Autodesk Fusion 360 part; units mm, degrees
(part 3 of 3)
  point P284 (15.4508, 47.5528)
  point P285 (-0.5155, 69.5286)
  point P286 (-5, 67.1945)
  point P287 (10.0646, 54.9663)
  point P288 (50, 67.9421)
  point P289 (39.8583, 55.4833)
  point P290 (50, 69.4421)
  point P291 (55, 67.1945)
  point P292 (43.541, 51.4226)
  point P293 (98.1857, -14.3619)
  point P294 (105.9017, -18.1636)
  point P295 (99.4427, -25.5195)
  point P296 (99.4698, -11.8417)
  point P297 (97.1866, -20.9953)
  point P298 (89.9352, -18.0941)
  point P299 (91.7173, -33.287)
  point P300 (55.3862, 7.4135)
  point P301 (56.2679, 8.627)
  point P302 (50.9017, 9.7476)
  point P303 (80.0676, 26.5576)
  point P304 (80.9017, 31.5439)
  point P305 (66.4847, 14.1828)
  point P306 (80.9017, 0)
  point P307 (52.5861, 20.5725)
  point P308 (62.958, 9.3287)
  point P309 (65.9663, 21.9758)
  point P310 (62.3607, 25.5195)
  point P311 (65.0847, 20.7623)
  point P312 (81.4942, 26.094)
  point P313 (99.9017, 12)
  point P314 (97.9017, 14)
  point P315 (89.9352, 18.0941)
  point P316 (80.9017, 0)
  point P317 (115.9017, 0)
  point P318 (75.3603, 21.7783)
  point P319 (58.477, 1.4597)
  point P320 (84.2289, 19.9482)
  point P321 (71.3525, 29.3893)
  point P322 (50, 0)
  point P323 (72.8402, 20.4942)
  point P324 (95.76, 21.4588)
  point P325 (105.9017, 7.5)
  point P326 (55.3862, -7.4135)
  point P327 (58.9194, -1.3339)
  point P328 (72.5838, -20.8761)
  point P329 (71.3525, -29.3893)
  point P330 (75.3774, -21.3186)
  point P331 (62.958, -9.3287)
  point P332 (52.5861, -20.5725)
  point P333 (105.9017, -7.5)
  point P334 (84.2289, -19.9482)
  point P335 (66.4847, -14.1828)
  point P336 (50.9017, -9.7476)
  point P337 (65.0847, -20.7623)
  point P338 (65.9663, -21.9758)
  point P339 (80.9017, -31.5439)
  point P340 (110.9017, -9.7476)
  point P341 (91.7173, 33.287)
  point P342 (100.9017, -3)
  point P343 (80.0676, -26.5576)
  point P344 (105.9017, -9)
  point P345 (95.76, -21.4588)
  point P346 (81.4942, -26.094)
  point P347 (105.9017, 9)
  point P348 (62.3607, -25.5195)
  point P349 (97.1866, 20.9953)
  point P350 (99.4427, 25.5195)
  point P351 (56.2679, -8.627)
  dimension "d15" = -5
  dimension "d17" = 360
  dimension "d19" = 360
  dimension "d22" = 360
  constraint coincident L11.start origin
  constraint coincident S5 L10.start
  constraint horizontal L11
  constraint midpoint S10.start L13
  constraint coincident S10 L15.start
  constraint midpoint S12.start L19
  constraint midpoint S6.start L21
  constraint midpoint S2.start L23
  constraint midpoint S7.start L25
  constraint midpoint S13.start L27
  constraint midpoint S18.start L33
  constraint midpoint S8.start L38
  constraint midpoint S3.start L42
  constraint midpoint S5.start L44
  constraint midpoint S4.start L46
  constraint midpoint S14.start L49
  constraint midpoint S0.start L51
  constraint midpoint S15.start L56
  constraint midpoint S1.start L58
  constraint midpoint S17.start L60
  constraint midpoint S9.start L62
  constraint midpoint S19.start L65
  constraint midpoint S16.start L68
  constraint symmetric L11.start L1 P92
  constraint symmetric L0.start L1 L29.start
  constraint symmetric L0.end L1 L29.end
  constraint symmetric L2.start L1 L54.start
  constraint symmetric L2.end L1 L41.start
  constraint symmetric L3.end L1 L40.start
  constraint symmetric L1 L5.start L30.end
  constraint symmetric L1 L5.end L53.start
  constraint symmetric L1 L6.end L32.start
  constraint symmetric L1 L7.end L31.start
  constraint symmetric L1 L8.end L30.start
  constraint symmetric L1 S0.start S32.start
  constraint symmetric L1 L12.end L36.end
  constraint symmetric L1 P0 P82
  constraint symmetric L1 P1 P76
  constraint symmetric L1 S1.start S34.start
  constraint symmetric L1 P2 P93
  constraint symmetric L1 P3 P97
  constraint symmetric L1 P4 P91
  constraint symmetric L1 S2.start S22.start
  constraint symmetric L1 P5 P72
  constraint symmetric L1 P6 P114
  constraint symmetric L1 P7 P59
  constraint symmetric L1 S3.start S27.start
  constraint symmetric L1 P8 P69
  constraint symmetric L1 P9 P78
  constraint symmetric L1 P10 P77
  constraint symmetric L1 S4.start S29.start
  constraint symmetric L1 P11 P110
  constraint symmetric L1 P12 P83
  constraint symmetric L1 P13 P89
  constraint symmetric L1 S5.start S28.start
  constraint symmetric L1 L10.end L64.end
  constraint symmetric L1 P14 P99
  constraint symmetric L1 P15 P88
  constraint symmetric L1 L10.start L64.start
  constraint symmetric L1 S6.start S21.start
  constraint symmetric L1 P16 P98
  constraint symmetric L1 P17 P70
  constraint symmetric L1 P18 P95
  constraint symmetric L1 S7.start S23.start
  constraint symmetric L1 P19 P64
  constraint symmetric L1 P20 P63
  constraint symmetric L1 P21 P67
  constraint symmetric L1 S8.start S26.start
  constraint symmetric L1 P22 P100
  constraint symmetric L1 P23 P79
  constraint symmetric L1 P24 P68
  constraint symmetric L1 S9.start S36.start
  constraint symmetric L1 P25 P75
  constraint symmetric L1 P26 P71
  constraint symmetric L1 P27 P81
  constraint symmetric L1 L11.start P92
  constraint symmetric L1 L16.end L35.end
  constraint symmetric L1 L11.end L37.end
  constraint symmetric L1 L15.end L17.end
  constraint symmetric L1 L12.start L36.start
  constraint symmetric L1 S10.start S38.start
  constraint symmetric L1 P28 P108
  constraint symmetric L1 P29 P106
  constraint symmetric L1 P30 P73
  constraint symmetric L1 S11.start S30.start
  constraint symmetric L1 P31 P112
  constraint symmetric L1 P32 P105
  constraint symmetric L1 L13.start L18.start
  constraint symmetric L1 L13.end L18.end
  constraint symmetric L1 L14.start L48.start
  constraint symmetric L1 L14.end L48.end
  constraint symmetric L1 L15.start L17.start
  constraint symmetric L1 S12.start S20.start
  constraint symmetric L1 P33 P103
  constraint symmetric L1 P34 P113
  constraint symmetric L1 P35 P102
  constraint symmetric L1 S13.start S24.start
  constraint symmetric L1 P36 P107
  constraint symmetric L1 P37 P104
  constraint symmetric L1 P38 P109
  constraint symmetric L1 S14.start S31.start
  constraint symmetric L1 P39 P65
  constraint symmetric L1 P40 P115
  constraint symmetric L1 P41 P84
  constraint symmetric L1 S15.start S33.start
  constraint symmetric L1 P42 P96
  constraint symmetric L1 P43 P111
  constraint symmetric L1 P44 P101
  constraint symmetric L1 S16.start S39.start
  constraint symmetric L1 P45 P62
  constraint symmetric L1 P46 P58
  constraint symmetric L1 P47 P74
  constraint symmetric L1 S17.start S35.start
  constraint symmetric L1 P48 P60
  constraint symmetric L1 P49 P87
  constraint symmetric L1 P50 P57
  constraint symmetric L1 S18.start S25.start
  constraint symmetric L1 P51 P86
  constraint symmetric L1 P52 P80
  constraint symmetric L1 P53 P94
  constraint symmetric L1 S19.start S37.start
  constraint symmetric L1 P54 P85
  constraint symmetric L1 P55 P66
  constraint symmetric L1 P56 P61
  constraint symmetric L1 L19.start L20.start
  constraint symmetric L1 L19.end L20.end
  constraint symmetric L1 L21.start L22.start
  constraint symmetric L1 L21.end L22.end
  constraint symmetric L1 L23.start L24.start
  constraint symmetric L1 L23.end L24.end
  constraint symmetric L1 L25.start L26.start
  constraint symmetric L1 L25.end L26.end
  constraint symmetric L1 L27.start L28.start
  constraint symmetric L1 L27.end L28.end
  constraint symmetric L1 L33.start L34.start
  constraint symmetric L1 L33.end L34.end
  constraint symmetric L1 L38.start L39.start
  constraint symmetric L1 L38.end L39.end
  constraint symmetric L1 L42.start L43.start
  constraint symmetric L1 L42.end L43.end
  constraint symmetric L1 L44.start L45.start
  constraint symmetric L1 L44.end L45.end
  constraint symmetric L1 L46.start L47.start
  constraint symmetric L1 L46.end L47.end
  constraint symmetric L1 L49.start L50.start
  constraint symmetric L1 L49.end L50.end
  constraint symmetric L1 L51.start L52.start
  constraint symmetric L1 L51.end L52.end
  constraint symmetric L1 L56.start L57.start
  constraint symmetric L1 L56.end L57.end
  constraint symmetric L1 L58.start L59.start
  constraint symmetric L1 L58.end L59.end
  constraint symmetric L1 L60.start L61.start
  constraint symmetric L1 L60.end L61.end
  constraint symmetric L1 L62.start L63.start
  constraint symmetric L1 L62.end L63.end
  constraint symmetric L1 L65.start L66.start
  constraint symmetric L1 L65.end L66.end
  constraint symmetric L1 L68.start L69.start
  constraint symmetric L1 L68.end L69.end
  constraint symmetric L11.start L0 P147
  constraint symmetric L4.end L0 L116.end
  constraint symmetric L1.start L0 L29.end
  constraint symmetric L1.end L0 L121.start
  constraint symmetric L2.end L0 L119.start
  constraint symmetric L3.end L0 L116.start
  constraint symmetric L0 L5.start L122.start
  constraint symmetric L0 L5.end L120.start
  constraint symmetric L0 L6.end L118.start
  constraint symmetric L0 L7.end L117.start
  constraint symmetric L0 L8.end L117.end
  constraint symmetric L0 S0.start S50.start
  constraint symmetric L0 L12.end L98.end
  constraint symmetric L0 P0 P149
  constraint symmetric L0 P1 P166
  constraint symmetric L0 S1.start S56.start
  constraint symmetric L0 P2 P158
  constraint symmetric L0 P3 P160
  constraint symmetric L0 P4 P171
  constraint symmetric L0 S2.start S59.start
  constraint symmetric L0 P5 P174
  constraint symmetric L0 P6 P172
  constraint symmetric L0 P7 P173
  constraint symmetric L0 S3.start S54.start
  constraint symmetric L0 P8 P145
  constraint symmetric L0 P9 P146
  constraint symmetric L0 P10 P128
  constraint symmetric L0 S4.start S52.start
  constraint symmetric L0 P11 P155
  constraint symmetric L0 P12 P162
  constraint symmetric L0 P13 P144
  constraint symmetric L0 S5.start S47.start
  constraint symmetric L0 L10.end L96.end
  constraint symmetric L0 P14 P130
  constraint symmetric L0 P15 P134
  constraint symmetric L0 L10.start L96.start
  constraint symmetric L0 S6.start S57.start
  constraint symmetric L0 P16 P132
  constraint symmetric L0 P17 P131
  constraint symmetric L0 P18 P135
  constraint symmetric L0 S7.start S58.start
  constraint symmetric L0 P19 P170
  constraint symmetric L0 P20 P123
  constraint symmetric L0 P21 P119
  constraint symmetric L0 S8.start S45.start
  constraint symmetric L0 P22 P148
  constraint symmetric L0 P23 P150
  constraint symmetric L0 P24 P151
  constraint symmetric L0 S9.start S46.start
  constraint symmetric L0 P25 P157
  constraint symmetric L0 P26 P154
  constraint symmetric L0 P27 P152
  constraint symmetric L0 L11.start P147
  constraint symmetric L0 L16.end L104.end
  constraint symmetric L0 L11.end L99.end
  constraint symmetric L0 L15.end L104.start
  constraint symmetric L0 L12.start L98.start
  constraint symmetric L0 S10.start S44.start
  constraint symmetric L0 P28 P138
  constraint symmetric L0 P29 P142
  constraint symmetric L0 P30 P136
  constraint symmetric L0 S11.start S53.start
  constraint symmetric L0 P31 P139
  constraint symmetric L0 P32 P133
  constraint symmetric L0 L13.start L83.start
  constraint symmetric L0 L13.end L83.end
  constraint symmetric L0 L14.start L106.start
  constraint symmetric L0 L14.end L106.end
  constraint symmetric L0 L15.start L105.start
  constraint symmetric L0 S12.start S41.start
  constraint symmetric L0 P33 P141
  constraint symmetric L0 P34 P164
  constraint symmetric L0 P35 P159
  constraint symmetric L0 S13.start S42.start
  constraint symmetric L0 P36 P169
  constraint symmetric L0 P37 P156
  constraint symmetric L0 P38 P165
  constraint symmetric L0 S14.start S55.start
  constraint symmetric L0 P39 P120
  constraint symmetric L0 P40 P121
  constraint symmetric L0 P41 P122
  constraint symmetric L0 S15.start S43.start
  constraint symmetric L0 P42 P126
  constraint symmetric L0 P43 P127
  constraint symmetric L0 P44 P125
  constraint symmetric L0 S16.start S48.start
  constraint symmetric L0 P45 P167
  constraint symmetric L0 P46 P168
  constraint symmetric L0 P47 P153
  constraint symmetric L0 S17.start S40.start
  constraint symmetric L0 P48 P124
  constraint symmetric L0 P49 P117
  constraint symmetric L0 P50 P116
  constraint symmetric L0 S18.start S51.start
  constraint symmetric L0 P51 P163
  constraint symmetric L0 P52 P129
  constraint symmetric L0 P53 P140
  constraint symmetric L0 S19.start S49.start
  constraint symmetric L0 P54 P143
  constraint symmetric L0 P55 P137
  constraint symmetric L0 P56 P161
  constraint symmetric L0 L19.start L77.start
  constraint symmetric L0 L19.end L77.end
  constraint symmetric L0 L21.start L80.start
  constraint symmetric L0 L21.end L80.end
  constraint symmetric L0 L23.start L103.start
  constraint symmetric L0 L23.end L103.end
  constraint symmetric L0 L25.start L74.start
  constraint symmetric L0 L25.end L74.end
  constraint symmetric L0 L27.start L78.start
  constraint symmetric L0 L27.end L78.end
  constraint symmetric L0 L33.start L82.start
  constraint symmetric L0 L33.end L82.end
  constraint symmetric L0 L38.start L84.start
  constraint symmetric L0 L38.end L84.end
  constraint symmetric L0 L42.start L88.start
  constraint symmetric L0 L42.end L88.end
  constraint symmetric L0 L44.start L85.start
  constraint symmetric L0 L44.end L85.end
  constraint symmetric L0 L46.start L100.start
  constraint symmetric L0 L46.end L100.end
  constraint symmetric L0 L49.start L75.start
  constraint symmetric L0 L49.end L75.end
  constraint symmetric L0 L51.start L94.start
  constraint symmetric L0 L51.end L94.end
  constraint symmetric L0 L56.start L71.start
  constraint symmetric L0 L56.end L71.end
  constraint symmetric L0 L58.start L73.start
  constraint symmetric L0 L58.end L73.end
  constraint symmetric L0 L60.start L72.start
  constraint symmetric L0 L60.end L72.end
  constraint symmetric L0 L62.start L86.start
  constraint symmetric L0 L62.end L86.end
  constraint symmetric L0 L65.start L93.start
  constraint symmetric L0 L65.end L93.end
  constraint symmetric L0 L68.start L89.start
  constraint symmetric L0 L68.end L89.end
  constraint symmetric L11.start L4 P202
  constraint symmetric L0.start L4 L116.end
  constraint symmetric L0.end L4 L135.end
  constraint symmetric L1.end L4 L136.start
  constraint symmetric L2.end L4 L136.end
  constraint symmetric L3.end L4 L138.end
  constraint symmetric L4 L5.start L155.start
  constraint symmetric L4 L5.end L139.start
  constraint symmetric L4 L6.end L139.end
  constraint symmetric L4 L7.end L126.start
  constraint symmetric L4 L8.end L126.end
  constraint symmetric L4 S0.start S78.start
  constraint symmetric L4 L12.end L137.end
  constraint symmetric L4 P0 P224
  constraint symmetric L4 P1 P223
  constraint symmetric L4 S1.start S66.start
  constraint symmetric L4 P2 P231
  constraint symmetric L4 P3 P225
  constraint symmetric L4 P4 P193
  constraint symmetric L4 S2.start S72.start
  constraint symmetric L4 P5 P190
  constraint symmetric L4 P6 P201
  constraint symmetric L4 P7 P197
  constraint symmetric L4 S3.start S77.start
  constraint symmetric L4 P8 P185
  constraint symmetric L4 P9 P186
  constraint symmetric L4 P10 P178
  constraint symmetric L4 S4.start S69.start
  constraint symmetric L4 P11 P179
  constraint symmetric L4 P12 P212
  constraint symmetric L4 P13 P232
  constraint symmetric L4 S5.start S76.start
  constraint symmetric L4 L10.end L163.end
  constraint symmetric L4 P14 P216
  constraint symmetric L4 P15 P228
  constraint symmetric L4 L10.start L163.start
  constraint symmetric L4 S6.start S73.start
  constraint symmetric L4 P16 P217
  constraint symmetric L4 P17 P222
  constraint symmetric L4 P18 P218
  constraint symmetric L4 S7.start S67.start
  constraint symmetric L4 P19 P192
  constraint symmetric L4 P20 P194
  constraint symmetric L4 P21 P195
  constraint symmetric L4 S8.start S74.start
  constraint symmetric L4 P22 P177
  constraint symmetric L4 P23 P176
  constraint symmetric L4 P24 P180
  constraint symmetric L4 S9.start S60.start
  constraint symmetric L4 P25 P181
  constraint symmetric L4 P26 P182
  constraint symmetric L4 P27 P175
  constraint symmetric L4 L11.start P202
  constraint symmetric L4 L16.end L132.end
  constraint symmetric L4 L11.end L167.end
  constraint symmetric L4 L15.end L125.end
  constraint symmetric L4 L12.start L137.start
  constraint symmetric L4 S10.start S75.start
  constraint symmetric L4 P28 P215
  constraint symmetric L4 P29 P213
  constraint symmetric L4 P30 P227
  constraint symmetric L4 S11.start S79.start
  constraint symmetric L4 P31 P220
  constraint symmetric L4 P32 P229
  constraint symmetric L4 L13.start L166.start
  constraint symmetric L4 L13.end L166.end
  constraint symmetric L4 L14.start L130.start
  constraint symmetric L4 L14.end L130.end
  constraint symmetric L4 L15.start L125.start
  constraint symmetric L4 S12.start S71.start
  constraint symmetric L4 P33 P226
  constraint symmetric L4 P34 P230
  constraint symmetric L4 P35 P233
  constraint symmetric L4 S13.start S70.start
  constraint symmetric L4 P36 P219
  constraint symmetric L4 P37 P214
  constraint symmetric L4 P38 P221
  constraint symmetric L4 S14.start S68.start
  constraint symmetric L4 P39 P187
  constraint symmetric L4 P40 P188
  constraint symmetric L4 P41 P189
  constraint symmetric L4 S15.start S65.start
  constraint symmetric L4 P42 P191
  constraint symmetric L4 P43 P198
  constraint symmetric L4 P44 P196
  constraint symmetric L4 S16.start S63.start
  constraint symmetric L4 P45 P207
  constraint symmetric L4 P46 P203
  constraint symmetric L4 P47 P208
  constraint symmetric L4 S17.start S64.start
  constraint symmetric L4 P48 P199
  constraint symmetric L4 P49 P200
  constraint symmetric L4 P50 P183
  constraint symmetric L4 S18.start S61.start
  constraint symmetric L4 P51 P204
  constraint symmetric L4 P52 P209
  constraint symmetric L4 P53 P211
  constraint symmetric L4 S19.start S62.start
  constraint symmetric L4 P54 P205
  constraint symmetric L4 P55 P210
  constraint symmetric L4 P56 P206
  constraint symmetric L4 L19.start L157.start
  constraint symmetric L4 L19.end L157.end
  constraint symmetric L4 L21.start L160.start
  constraint symmetric L4 L21.end L160.end
  constraint symmetric L4 L23.start L159.start
  constraint symmetric L4 L23.end L159.end
  constraint symmetric L4 L25.start L147.start
  constraint symmetric L4 L25.end L147.end
  constraint symmetric L4 L27.start L152.start
  constraint symmetric L4 L27.end L152.end
  constraint symmetric L4 L33.start L133.start
  constraint symmetric L4 L33.end L133.end
  constraint symmetric L4 L38.start L127.start
  constraint symmetric L4 L38.end L127.end
  constraint symmetric L4 L42.start L134.start
  constraint symmetric L4 L42.end L134.end
  constraint symmetric L4 L44.start L169.start
  constraint symmetric L4 L44.end L169.end
  constraint symmetric L4 L46.start L129.start
  constraint symmetric L4 L46.end L129.end
  constraint symmetric L4 L49.start L150.start
  constraint symmetric L4 L49.end L150.end
  constraint symmetric L4 L51.start L170.start
  constraint symmetric L4 L51.end L170.end
  constraint symmetric L4 L56.start L143.start
  constraint symmetric L4 L56.end L143.end
  constraint symmetric L4 L58.start L144.start
  constraint symmetric L4 L58.end L144.end
  constraint symmetric L4 L60.start L142.start
  constraint symmetric L4 L60.end L142.end
  constraint symmetric L4 L62.start L128.start
  constraint symmetric L4 L62.end L128.end
  constraint symmetric L4 L65.start L140.start
  constraint symmetric L4 L65.end L140.end
  constraint symmetric L4 L68.start L141.start
  constraint symmetric L4 L68.end L141.end
  constraint symmetric L11.start L3 P273
  constraint symmetric L0.start L3 L224.end
  constraint symmetric L0.end L3 L208.start
  constraint symmetric L1.end L3 L208.end
  constraint symmetric L2.end L3 L231.end
  constraint symmetric L4.start L3 L138.end
  constraint symmetric L3 L5.start L216.start
  constraint symmetric L3 L5.end L206.start
  constraint symmetric L3 L6.end L193.start
  constraint symmetric L3 L7.end L182.start
  constraint symmetric L3 L8.end L182.end
  constraint symmetric L3 S0.start S97.start
  constraint symmetric L3 L12.end L227.end
  constraint symmetric L3 P0 P277
  constraint symmetric L3 P1 P264
  constraint symmetric L3 S1.start S89.start
  constraint symmetric L3 P2 P275
  constraint symmetric L3 P3 P261
  constraint symmetric L3 P4 P274
  constraint symmetric L3 S2.start S92.start
  constraint symmetric L3 P5 P247
  constraint symmetric L3 P6 P244
  constraint symmetric L3 P7 P237
  constraint symmetric L3 S3.start S83.start
  constraint symmetric L3 P8 P238
  constraint symmetric L3 P9 P266
  constraint symmetric L3 P10 P279
  constraint symmetric L3 S4.start S99.start
  constraint symmetric L3 P11 P281
  constraint symmetric L3 P12 P280
  constraint symmetric L3 P13 P282
  constraint symmetric L3 S5.start S82.start
  constraint symmetric L3 L10.end L188.end
  constraint symmetric L3 P14 P283
  constraint symmetric L3 P15 P267
  constraint symmetric L3 L10.start L188.start
  constraint symmetric L3 S6.start S90.start
  constraint symmetric L3 P16 P265
  constraint symmetric L3 P17 P262
  constraint symmetric L3 P18 P251
  constraint symmetric L3 S7.start S91.start
  constraint symmetric L3 P19 P240
  constraint symmetric L3 P20 P271
  constraint symmetric L3 P21 P239
  constraint symmetric L3 S8.start S86.start
  constraint symmetric L3 P22 P242
  constraint symmetric L3 P23 P243
  constraint symmetric L3 P24 P241
  constraint symmetric L3 S9.start S80.start
  constraint symmetric L3 P25 P260
  constraint symmetric L3 P26 P284
  constraint symmetric L3 P27 P268
  constraint symmetric L3 L11.start P273
  constraint symmetric L3 L16.end L226.end
  constraint symmetric L3 L11.end L194.end
  constraint symmetric L3 L15.end L226.start
  constraint symmetric L3 L12.start L227.start
  constraint symmetric L3 S10.start S98.start
  constraint symmetric L3 P28 P250
  constraint symmetric L3 P29 P248
  constraint symmetric L3 P30 P285
  constraint symmetric L3 S11.start S81.start
  constraint symmetric L3 P31 P286
  constraint symmetric L3 P32 P269
  constraint symmetric L3 L13.start L219.start
  constraint symmetric L3 L13.end L219.end
  constraint symmetric L3 L14.start L184.start
  constraint symmetric L3 L14.end L184.end
  constraint symmetric L3 L15.start L229.start
  constraint symmetric L3 S12.start S94.start
  constraint symmetric L3 P33 P253
  constraint symmetric L3 P34 P263
  constraint symmetric L3 P35 P249
  constraint symmetric L3 S13.start S95.start
  constraint symmetric L3 P36 P254
  constraint symmetric L3 P37 P246
  constraint symmetric L3 P38 P245
  constraint symmetric L3 S14.start S88.start
  constraint symmetric L3 P39 P236
  constraint symmetric L3 P40 P270
  constraint symmetric L3 P41 P235
  constraint symmetric L3 S15.start S93.start
  constraint symmetric L3 P42 P278
  constraint symmetric L3 P43 P276
  constraint symmetric L3 P44 P272
  constraint symmetric L3 S16.start S87.start
  constraint symmetric L3 P45 P234
  constraint symmetric L3 P46 P292
  constraint symmetric L3 P47 P289
  constraint symmetric L3 S17.start S96.start
  constraint symmetric L3 P48 P288
  constraint symmetric L3 P49 P291
  constraint symmetric L3 P50 P290
  constraint symmetric L3 S18.start S84.start
  constraint symmetric L3 P51 P287
  constraint symmetric L3 P52 P256
  constraint symmetric L3 P53 P255
  constraint symmetric L3 S19.start S85.start
  constraint symmetric L3 P54 P259
  constraint symmetric L3 P55 P258
  constraint symmetric L3 P56 P257
  constraint symmetric L3 L19.start L202.start
  constraint symmetric L3 L19.end L202.end
  constraint symmetric L3 L21.start L200.start
  constraint symmetric L3 L21.end L200.end
  constraint symmetric L3 L23.start L210.start
  constraint symmetric L3 L23.end L210.end
  constraint symmetric L3 L25.start L209.start
  constraint symmetric L3 L25.end L209.end
  constraint symmetric L3 L27.start L215.start
  constraint symmetric L3 L27.end L215.end
  constraint symmetric L3 L33.start L190.start
  constraint symmetric L3 L33.end L190.end
  constraint symmetric L3 L38.start L197.start
  constraint symmetric L3 L38.end L197.end
  constraint symmetric L3 L42.start L181.start
  constraint symmetric L3 L42.end L181.end
  constraint symmetric L3 L44.start L191.start
  constraint symmetric L3 L44.end L191.end
  constraint symmetric L3 L46.start L186.start
  constraint symmetric L3 L46.end L186.end
  constraint symmetric L3 L49.start L199.start
  constraint symmetric L3 L49.end L199.end
  constraint symmetric L3 L51.start L187.start
  constraint symmetric L3 L51.end L187.end
  constraint symmetric L3 L56.start L203.start
  constraint symmetric L3 L56.end L203.end
  constraint symmetric L3 L58.start L204.start
  constraint symmetric L3 L58.end L204.end
  constraint symmetric L3 L60.start L207.start
  constraint symmetric L3 L60.end L207.end
  constraint symmetric L3 L62.start L180.start
  constraint symmetric L3 L62.end L180.end
  constraint symmetric L3 L65.start L185.start
  constraint symmetric L3 L65.end L185.end
  constraint symmetric L3 L68.start L179.start
  constraint symmetric L3 L68.end L179.end
  constraint symmetric L11.start L2 P316
  constraint symmetric L0.start L2 L251.start
  constraint symmetric L0.end L2 L251.end
  constraint symmetric L1.end L2 L54.start
  constraint symmetric L3.start L2 L231.end
  constraint symmetric L3.end L2 L252.start
  constraint symmetric L2 L5.start L248.end
  constraint symmetric L2 L5.end L274.end
  constraint symmetric L2 L6.end L256.start
  constraint symmetric L2 L7.end L254.start
  constraint symmetric L2 L8.end L248.start
  constraint symmetric L2 S0.start S111.start
  constraint symmetric L2 L12.end L239.end
  constraint symmetric L2 P0 P317
  constraint symmetric L2 P1 P342
  constraint symmetric L2 S1.start S115.start
  constraint symmetric L2 P2 P298
  constraint symmetric L2 P3 P299
  constraint symmetric L2 P4 P334
  constraint symmetric L2 S2.start S118.start
  constraint symmetric L2 P5 P335
  constraint symmetric L2 P6 P332
  constraint symmetric L2 P7 P331
  constraint symmetric L2 S3.start S100.start
  constraint symmetric L2 P8 P308
  constraint symmetric L2 P9 P307
  constraint symmetric L2 P10 P305
  constraint symmetric L2 S4.start S108.start
  constraint symmetric L2 P11 P320
  constraint symmetric L2 P12 P341
  constraint symmetric L2 P13 P315
  constraint symmetric L2 S5.start S109.start
  constraint symmetric L2 L10.end L240.end
  constraint symmetric L2 P14 P314
  constraint symmetric L2 P15 P313
  constraint symmetric L2 L10.start L240.start
  constraint symmetric L2 S6.start S114.start
  constraint symmetric L2 P16 P296
  constraint symmetric L2 P17 P294
  constraint symmetric L2 P18 P293
  constraint symmetric L2 S7.start S117.start
  constraint symmetric L2 P19 P330
  constraint symmetric L2 P20 P329
  constraint symmetric L2 P21 P328
  constraint symmetric L2 S8.start S105.start
  constraint symmetric L2 P22 P327
  constraint symmetric L2 P23 P322
  constraint symmetric L2 P24 P319
  constraint symmetric L2 S9.start S102.start
  constraint symmetric L2 P25 P323
  constraint symmetric L2 P26 P321
  constraint symmetric L2 P27 P318
  constraint symmetric L2 L11.start P316
  constraint symmetric L2 L16.end L257.end
  constraint symmetric L2 L11.end L258.end
  constraint symmetric L2 L15.end L243.end
  constraint symmetric L2 L12.start L239.start
  constraint symmetric L2 S10.start S103.start
  constraint symmetric L2 P28 P347
  constraint symmetric L2 P29 P325
  constraint symmetric L2 P30 P349
  constraint symmetric L2 S11.start S101.start
  constraint symmetric L2 P31 P350
  constraint symmetric L2 P32 P324
  constraint symmetric L2 L13.start L238.start
  constraint symmetric L2 L13.end L238.end
  constraint symmetric L2 L14.start L234.start
  constraint symmetric L2 L14.end L234.end
  constraint symmetric L2 L15.start L243.start
  constraint symmetric L2 S12.start S119.start
  constraint symmetric L2 P33 P297
  constraint symmetric L2 P34 P295
  constraint symmetric L2 P35 P345
  constraint symmetric L2 S13.start S116.start
  constraint symmetric L2 P36 P344
  constraint symmetric L2 P37 P340
  constraint symmetric L2 P38 P333
  constraint symmetric L2 S14.start S113.start
  constraint symmetric L2 P39 P338
  constraint symmetric L2 P40 P348
  constraint symmetric L2 P41 P337
  constraint symmetric L2 S15.start S112.start
  constraint symmetric L2 P42 P343
  constraint symmetric L2 P43 P339
  constraint symmetric L2 P44 P346
  constraint symmetric L2 S16.start S106.start
  constraint symmetric L2 P45 P300
  constraint symmetric L2 P46 P302
  constraint symmetric L2 P47 P301
  constraint symmetric L2 S17.start S110.start
  constraint symmetric L2 P48 P326
  constraint symmetric L2 P49 P336
  constraint symmetric L2 P50 P351
  constraint symmetric L2 S18.start S104.start
  constraint symmetric L2 P51 P303
  constraint symmetric L2 P52 P304
  constraint symmetric L2 P53 P312
  constraint symmetric L2 S19.start S107.start
  constraint symmetric L2 P54 P309
  constraint symmetric L2 P55 P310
  constraint symmetric L2 P56 P311
  constraint symmetric L2 L19.start L278.start
  constraint symmetric L2 L19.end L278.end
  constraint symmetric L2 L21.start L272.start
  constraint symmetric L2 L21.end L272.end
  constraint symmetric L2 L23.start L271.start
  constraint symmetric L2 L23.end L271.end
  constraint symmetric L2 L25.start L280.start
  constraint symmetric L2 L25.end L280.end
  constraint symmetric L2 L27.start L275.start
  constraint symmetric L2 L27.end L275.end
  constraint symmetric L2 L33.start L242.start
  constraint symmetric L2 L33.end L242.end
  constraint symmetric L2 L38.start L244.start
  constraint symmetric L2 L38.end L244.end
  constraint symmetric L2 L42.start L233.start
  constraint symmetric L2 L42.end L233.end
  constraint symmetric L2 L44.start L247.start
  constraint symmetric L2 L44.end L247.end
  constraint symmetric L2 L46.start L237.start
  constraint symmetric L2 L46.end L237.end
  constraint symmetric L2 L49.start L269.start
  constraint symmetric L2 L49.end L269.end
  constraint symmetric L2 L51.start L261.start
  constraint symmetric L2 L51.end L261.end
  constraint symmetric L2 L56.start L268.start
  constraint symmetric L2 L56.end L268.end
  constraint symmetric L2 L58.start L266.start
  constraint symmetric L2 L58.end L266.end
  constraint symmetric L2 L60.start L265.start
  constraint symmetric L2 L60.end L265.end
  constraint symmetric L2 L62.start L235.start
  constraint symmetric L2 L62.end L235.end
  constraint symmetric L2 L65.start L236.start
  constraint symmetric L2 L65.end L236.end
  constraint symmetric L2 L68.start L249.start
  constraint symmetric L2 L68.end L249.end
extrude "Extrude1" add sketch "Sketch1" along normal blind 2 contours L5 L6 L7 L8 L9 | L30 L31 L32 L53 L55 | L117 L118 L120 L122 L123 | L126 L139 L155 L164 L176 | L182 L193 L206 L216 L223 | L248 L254 L256 L274 L284 makes body 1 at (14.5324, 0, 44.6641) makes body 2 at (10.504, 0, 32.2661) makes body 3 at (70.3977, 0, 32.2661) makes body 4 at (-37.9874, 0, 27.6231) makes body 5 at (-75.9185, 0, -79.8308) makes body 6 at (52.4635, 0, -96.8718)
extrude "Extrude2" add sketch "Sketch1" along normal blind 3 contours L4 L135 L136 L138 L149 bodies 5
extrude "Extrude3" add sketch "Sketch1" along normal blind 3 contours L3 L208 L224 L225 L231 bodies 6
extrude "Extrude4" add sketch "Sketch1" along normal blind 3 contours L2 L251 L252 L253 L277 bodies 3
extrude "Extrude5" add sketch "Sketch1" along normal blind 3 contours L0 L116 L119 L121 L124 bodies 4
extrude "Extrude6" add sketch "Sketch1" along normal blind 3 contours L0 L1 L2 L3 L4 bodies 2
extrude "Extrude7" add sketch "Sketch1" along normal blind 3 contours L1 L29 L40 L41 L54 bodies 1
move_body "Move1" bodies 4 to x (0.730202, 0.654508, 0.19602) y (-0.654508, 0.587785, 0.475528) z (0.19602, -0.475528, 0.857583) at (-13.4899, 32.7254, 9.801)
move_body "Move2" bodies 5 to x (0.730202, 0.654508, -0.19602) y (-0.654508, 0.587785, -0.475528) z (-0.19602, 0.475528, 0.857583) at (-13.4899, 32.7254, -9.801)
move_body "Move3" bodies 4 to x (0.996415, 0.084565, 0.002605) y (-0.084565, 0.994522, 0.06144) z (0.002605, -0.06144, 0.998107) at (-0.1793, 4.2283, 0.1302)
move_body "Move4" bodies 5 to x (0.996415, 0.084565, -0.002605) y (-0.084565, 0.994522, -0.06144) z (-0.002605, 0.06144, 0.998107) at (-0.1793, 4.2283, -0.1302)
move_body "Move5" bodies 4 to x (0.999601, 0.028234, 0.00029) y (-0.028234, 0.999391, 0.020513) z (0.00029, -0.020513, 0.99979) at (-0.0199, 1.4117, 0.0145)
move_body "Move6" bodies 5 to x (0.999601, 0.028234, -0.00029) y (-0.028234, 0.999391, -0.020513) z (-0.00029, 0.020513, 0.99979) at (-0.0199, 1.4117, -0.0145)
move_body "Move7" bodies 4 to x (0.9999, 0.014119, 0.000072) y (-0.014119, 0.999848, 0.010258) z (0.000072, -0.010258, 0.999947) at (-0.005, 0.706, 0.0036)
move_body "Move8" bodies 5 to x (0.999601, 0.028234, -0.00029) y (-0.028234, 0.999391, -0.020513) z (-0.00029, 0.020513, 0.99979) at (-0.0199, 1.4117, -0.0145)
move_body "Move9" bodies 4 to x (0.9999, 0.014119, 0.000072) y (-0.014119, 0.999848, 0.010258) z (0.000072, -0.010258, 0.999947) at (-0.005, 0.706, 0.0036)
move_body "Move10" bodies 6 to x (0.946369, -0.277743, 0.165059) y (0.277743, 0.438371, -0.854804) z (0.165059, 0.854804, 0.492002) at (7.0204, 36.357, -21.6064)
move_body "Move11" bodies 3 to x (0.438371, -0.898794, 0) y (0.898794, 0.438371, 0) z (0, 0, 1) at (22.7184, 36.357, 0)
move_body "Move12" bodies 1 to x (0.946369, -0.277743, -0.165059) y (0.277743, 0.438371, 0.854804) z (-0.165059, -0.854804, 0.492002) at (7.0204, 36.357, 21.6064)
mirror "Mirror1" about plane through (24.7528, -81.2967, 76.1814) normal (-0.449424, -0.72714, 0.518928) of bodies 1 makes body 7
move_body "Move13" bodies 7 to x (0.847596, -0.249316, 0.468425) y (-0.240507, 0.606381, 0.75793) z (-0.473008, -0.755079, 0.454004) at (20.2544, 31.6943, 91.6171)
mirror "Mirror2" about plane through (80.1019, -81.2967, 0) normal (0.35465, -0.72714, 0.587785) of bodies 3 makes body 8
move_body "Move14" bodies 8 to x (0.490242, -0.795165, 0.356897) y (0.646514, 0.606381, 0.462949) z (-0.584537, 0.003782, 0.811358) at (93.392, 31.6943, 9.0481)
mirror "Mirror3" about plane through (24.7528, -81.2967, -76.1814) normal (0.66861, -0.72714, -0.155656) of bodies 6 makes body 9
move_body "Move15" bodies 9 to x (0.713793, -0.242123, 0.657173) y (0.640075, 0.606381, -0.471812) z (-0.284261, 0.757416, 0.587807) at (37.465, 31.6943, -86.0251)
mirror "Mirror4" about plane through (-64.8038, -81.2967, -47.0827) normal (0.058574, -0.72714, -0.683986) of bodies 5 makes body 10
move_body "Move16" bodies 10 to x (0.709434, 0.645525, 0.282844) y (-0.250926, 0.606381, -0.754545) z (-0.658589, 0.464327, 0.592166) at (-70.2374, 31.6943, -62.2146)
mirror "Mirror5" about plane through (-64.8038, -81.2967, 47.0827) normal (-0.632409, -0.72714, -0.26707) of bodies 4 makes body 11
move_body "Move17" bodies 11 to x (0.492935, 0.641079, 0.588245) y (-0.795155, 0.606381, 0.005477) z (-0.353189, -0.470446, 0.808664) at (-80.8741, 31.6943, 47.5744)
move_body "Move18" bodies 7 2 9 8 11 1 3 4 6 5 10 to x (1, 0, 0) y (0, 1, 0) z (0, 0, 1) at (0, 133, 0)
sketch "Sketch6" plane through (0, 0, 0) normal (0, 1, 0) x (1, 0, 0)
  line L0 (0, 0) -> (0, -45)
  line L1 (0, 0) -> (0, 45)
  arc A0 (0, -45) -> (0, 45) centre (0, 0) ccw
  dimension "d48" = 45
  constraint coincident L0.start L1.start
  constraint vertical L0
  constraint parallel L0 L1
  measures "d48" distance of L0.start L1.end
revolve "Revolve1" add sketch "Sketch6" angle 360 about axis through (0, 0, 0) along (0, 0, -1) separate body makes body 12
move_body "Move19" bodies 12 to x (1, 0, 0) y (0, 1, 0) z (0, 0, 1) at (0, 60, 0)
hidden bodies 12
